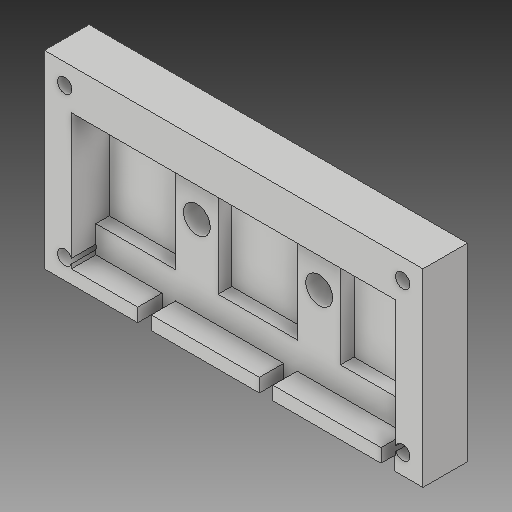
# Autodesk Inventor part: ArduinPanelRelay
Saved by Autodesk Inventor 2018 (Build 220112000, 112)
## iProperties
Created: 2020-04-10
Part Number: ArduinPanelRelay
Material: Generic
Document SubType Name: Modeling
Designer: emile
Density: 1 g/cm^3
Appearance: Default
Mass: 177.561 g
Surface Area: 527.277 cm^2
Volume: 177.561 cm^3
Author: emile
Autodesk Inventor part; units mm, degrees
ref_plane "YZ Plane" through (0, 0, 0) normal (1, 0, 0) x (0, 1, 0)
ref_plane "XZ Plane" through (0, 0, 0) normal (0, 1, 0) x (-1, 0, 0)
ref_plane "XY Plane" through (0, 0, 0) normal (0, 0, 1) x (1, 0, 0)
sketch "Sketch1" plane through (0, 0, 0) normal (0, 0, 1) x (1, 0, 0)
  line L0 (88.9, -44.45) -> (-88.9, -44.45)
  line L1 (-88.9, -44.45) -> (-88.9, 44.45)
  line L2 (-88.9, 44.45) -> (88.9, 44.45)
  line L3 (88.9, 44.45) -> (88.9, -44.45)
  line L4 (88.9, -44.45) -> (-88.9, 44.45) construction
  line L5 (-88.9, -44.45) -> (88.9, 44.45) construction
  line L6 (-38.735, -25.4) -> (-76.2, -25.4)
  line L7 (-76.2, -25.4) -> (-76.2, 25.4)
  line L8 (-76.2, 25.4) -> (-38.735, 25.4)
  line L9 (-38.735, 25.4) -> (-38.735, -25.4)
  line L10 (-38.735, -25.4) -> (-76.2, 25.4) construction
  line L11 (-76.2, -25.4) -> (-38.735, 25.4) construction
  line L12 (18.7325, -25.4) -> (-18.7325, -25.4)
  line L13 (-18.7325, -25.4) -> (-18.7325, 25.4)
  line L14 (-18.7325, 25.4) -> (18.7325, 25.4)
  line L15 (18.7325, 25.4) -> (18.7325, -25.4)
  line L16 (18.7325, -25.4) -> (-18.7325, 25.4) construction
  line L17 (-18.7325, -25.4) -> (18.7325, 25.4) construction
  line L18 (76.2, -25.4) -> (38.735, -25.4)
  line L19 (38.735, -25.4) -> (38.735, 25.4)
  line L20 (38.735, 25.4) -> (76.2, 25.4)
  line L21 (76.2, 25.4) -> (76.2, -25.4)
  line L22 (76.2, -25.4) -> (38.735, 25.4) construction
  line L23 (38.735, -25.4) -> (76.2, 25.4) construction
  line L24 (-38.735, 25.4) -> (-38.735, -25.4)
  line L25 (-38.735, -25.4) -> (-18.7325, -25.4)
  line L26 (-18.7325, -25.4) -> (-18.7325, 25.4)
  line L27 (-18.7325, 25.4) -> (-38.735, 25.4)
  line L28 (18.7325, 25.4) -> (18.7325, -25.4)
  line L29 (18.7325, -25.4) -> (38.735, -25.4)
  line L30 (38.735, -25.4) -> (38.735, 25.4)
  line L31 (38.735, 25.4) -> (18.7325, 25.4)
  line L32 (-76.2, -25.4) -> (76.2, -25.4)
  line L33 (76.2, -25.4) -> (76.2, -38.1)
  line L34 (76.2, -38.1) -> (-76.2, -38.1)
  line L35 (-76.2, -38.1) -> (-76.2, -25.4)
  point P0 (0, 0)
  point P1 (-57.4675, 0)
  point P2 (-57.4675, 0)
  point P3 (0, 0)
  point P4 (57.4675, 0)
  point P5 (0, 0)
  point P6 (57.4675, 0)
  dimension "d0" = 177.8
  dimension "d1" = 88.9
  dimension "d2" = 37.465
  dimension "d3" = 50.8
  dimension "d4" = 12.7
  dimension "d5" = 12.7
  dimension "d6" = 12.7
  constraints: 72 end point, 19 equal length, 12 midpoint, 9 perpendicular, 4 horizontal, 2 horizontal alignment
  measures "d0" distance of L1.end L2.end
  measures "d1" distance of L0.end L1.end
  measures "d2" distance of L7.end L8.end
  measures "d3" distance of L8.end L6.start
  measures "d4" distance between parallel lines of L1 L7
  measures "d5" distance between parallel lines of L3 L21
  measures "d6" distance between parallel lines of L32 L34
extrude "Extrusion1" add sketch "Sketch1" along normal blind 17.78
extrude "Extrusion2" add sketch "Sketch1" against normal blind 3.175 contours L0 L1 L2 L3 | L25 L12 L29 L18 L33 L34 L35 L6 | L6 L7 L8 L9 | L9 L27 L13 L25 | L13 L14 L15 L12 | L15 L31 L19 L29 | L19 L20 L21 L18
extrude "Extrusion3" add sketch "Sketch1" along normal blind 6.35 contours L25 L12 L29 L18 L33 L34 L35 L6 | L9 L27 L13 L25 | L15 L31 L19 L29
sketch "Sketch2" plane through (0, 0, 17.78) normal (0, 0, 1) x (1, 0, 0)
  line L0 (-38.735, -25.4) -> (-76.2, -25.4) projected
  line L1 (-38.735, -25.4) -> (-38.735, -44.45)
  line L2 (88.9, -44.45) -> (-88.9, -44.45) projected
  line L3 (-38.735, -44.45) -> (-45.085, -44.45)
  line L4 (76.2, -38.1) -> (-76.2, -38.1) projected
  line L5 (-45.085, -38.1) -> (-45.085, -44.45)
  line L6 (-45.085, -38.1) -> (-38.735, -38.1)
  point P0 (0, 0)
  dimension "d13" = 6.35
  constraints: 8 end point, 5 point on line, 1 perpendicular, 1 vertical
  measures "d13" distance between parallel lines of L1 L5
extrude "Extrusion4" cut sketch "Sketch2" against normal up to surface (11.43 mm away)
pattern_linear "Rectangular Pattern1" count 3 spacing 57.15 along (1, 0, 0) of "Extrusion4"
sketch "Sketch3" plane through (0, 0, -3.175) normal (0, 0, -1) x (-1, 0, 0)
  point P0 (-79.375, 34.925)
  point P1 (-79.375, -34.925)
  point P2 (79.375, -34.925)
  point P3 (79.375, 34.925)
hole "Hole1" at (79.375, 34.925, -3.175) at (79.375, -34.925, -3.175) at (-79.375, -34.925, -3.175) at (-79.375, 34.925, -3.175) direction (0, 0, 1) diameter 6.7564 depth 20.955
sketch "Sketch4" plane through (0, 0, 6.35) normal (0, 0, 1) x (1, 0, 0)
  arc A0 (-76.2, -36.079) -> (-76.2, -33.771) centre (-79.375, -34.925) ccw projected
  line L0 (-76.2, -38.1) -> (-76.2, -36.079) projected
  line L1 (-45.085, -38.1) -> (-76.2, -38.1) projected
  line L2 (-45.085, -44.45) -> (-45.085, -38.1) projected
  line L3 (-38.735, -44.45) -> (-45.085, -44.45) projected
  line L4 (-38.735, -38.1) -> (-38.735, -44.45) projected
  line L5 (12.065, -38.1) -> (-38.735, -38.1) projected
  line L6 (12.065, -44.45) -> (12.065, -38.1) projected
  line L7 (18.415, -44.45) -> (12.065, -44.45) projected
  line L8 (18.415, -38.1) -> (18.415, -44.45) projected
  line L9 (69.215, -38.1) -> (18.415, -38.1) projected
  line L10 (69.215, -44.45) -> (69.215, -38.1) projected
  line L11 (75.565, -44.45) -> (69.215, -44.45) projected
  line L12 (75.565, -38.1) -> (75.565, -44.45) projected
  line L13 (76.2, -38.1) -> (75.565, -38.1) projected
  line L14 (76.2, -36.079) -> (76.2, -38.1) projected
  arc A1 (76.2, -33.771) -> (76.2, -36.079) centre (79.375, -34.925) ccw projected
  line L15 (76.2, -25.4) -> (76.2, -33.771) projected
  line L16 (76.2, -25.4) -> (38.735, -25.4) projected
  line L17 (38.735, -25.4) -> (38.735, 25.4) projected
  line L18 (18.7325, 25.4) -> (38.735, 25.4) projected
  line L19 (18.7325, 25.4) -> (18.7325, -25.4) projected
  line L20 (18.7325, -25.4) -> (-18.7325, -25.4) projected
  line L21 (-18.7325, -25.4) -> (-18.7325, 25.4) projected
  line L22 (-38.735, 25.4) -> (-18.7325, 25.4) projected
  line L23 (-38.735, 25.4) -> (-38.735, -25.4) projected
  line L24 (-38.735, -25.4) -> (-76.2, -25.4) projected
  line L25 (-76.2, -33.771) -> (-76.2, -25.4) projected
  circle A2 centre (-28.7338, 0) radius 6.35
  circle A3 centre (28.7338, 0) radius 6.35
  point P0 (0, 0)
  point P1 (-28.7338, 25.4)
  point P2 (28.7338, 25.4)
  dimension "d26" = 12.7
  constraints: 2 centre point, 2 horizontal alignment, 2 midpoint, 2 vertical alignment, 1 equal radius
  measures "d26" diameter of A2
extrude "Extrusion5" cut sketch "Sketch4" against normal through all contours A2 | A3
equation "\"d5\" = d4"
body "Solid1"
